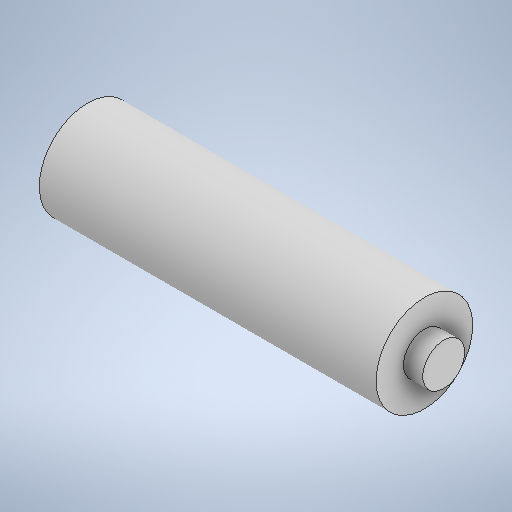
# Autodesk Inventor part: rodillo con rodamiento 2
Saved by Autodesk Inventor 2025 (Build 290162000, 162)
## iProperties
Created: 2026-09-21
Part Number: rodillo con rodamiento 2
Material: Genérico
Document SubType Name: Modeling
Designer: ASUS
Density: 1 g/cm^3
Appearance: Valor por defecto
Author: ASUS
Autodesk Inventor part; units mm, degrees
ref_plane "YZ Plane" through (0, 0, 0) normal (1, 0, 0) x (0, 1, 0)
ref_plane "XZ Plane" through (0, 0, 0) normal (0, 1, 0) x (-1, 0, 0)
ref_plane "XY Plane" through (0, 0, 0) normal (0, 0, 1) x (1, 0, 0)
sketch "Boceto1" plane through (0, 0, 0) normal (1, 0, 0) x (0, 1, 0)
  circle A0 centre (0, 0) radius 15
  dimension "d0" = 30
  constraints: 1 centre point, 1 coincident
  measures "d0" diameter of A0
extrude "Extrusión1" add sketch "Boceto1" along normal blind 104.547
sketch "Boceto2" plane through (104.547, 0, 0) normal (1, 0, 0) x (0, 0, -1)
  circle A0 centre (0, 0) radius 6.5
  dimension "d3" = 13
  constraints: 1 centre point, 1 coincident
  measures "d3" diameter of A0
extrude "Extrusión2" add sketch "Boceto2" along normal blind 6
sketch "Boceto3" plane through (0, 0, 0) normal (-1, 0, 0) x (0, 0, 1)
  circle A0 centre (0, 0) radius 6.5
  dimension "d6" = 13
  constraints: 1 centre point, 1 coincident
  measures "d6" diameter of A0
extrude "Extrusión3" add sketch "Boceto3" along normal blind 6
